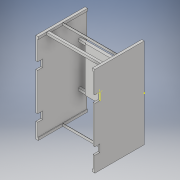
# Autodesk Inventor part: stand2.0
Saved by Autodesk Inventor 2019 (Build 230136000, 136)
## iProperties
Created: 2020-02-10
Part Number: stand2.0
Material: Generic
Document SubType Name: Modeling
Designer: Dell
Density: 1 g/cm^3
Appearance: Default
Author: Dell
Autodesk Inventor part; units mm, degrees
ref_plane "YZ Plane" through (0, 0, 0) normal (1, 0, 0) x (0, 1, 0)
ref_plane "XZ Plane" through (0, 0, 0) normal (0, 1, 0) x (-1, 0, 0)
ref_plane "XY Plane" through (0, 0, 0) normal (0, 0, 1) x (1, 0, 0)
sketch "Sketch1" plane through (0, 0, 0) normal (0, 0, 1) x (1, 0, 0)
  line L0 (-240, 365) -> (240, 365)
  line L1 (240, 365) -> (240, -365)
  line L2 (240, -365) -> (-240, -365)
  line L3 (-240, -365) -> (-240, 365)
  line L4 (-225, 345) -> (225, 345)
  line L5 (225, 345) -> (225, -345)
  line L6 (225, -345) -> (-225, -345)
  line L7 (-225, -345) -> (-225, 345)
  point P0 (0, 0)
  dimension "d0" = 480
  dimension "d1" = 730
  dimension "d2" = 450
  dimension "d3" = 690
  constraints: 16 end point, 4 parallel, 2 horizontal, 2 perpendicular
  measures "d0" distance of L1.end L2.end
  measures "d1" distance of L0.end L1.end
  measures "d2" distance of L5.end L6.end
  measures "d3" distance of L4.end L5.end
extrude "Extrusion1" add sketch "Sketch1" along normal blind 400
sketch "Sketch2" plane through (-240, 365, 0) normal (0, 1, 0) x (1, 0, 0)
  line L0 (20, 0) -> (20, -199)
  line L1 (20, 0) -> (219, 0) construction
  line L2 (20, -199) -> (460, -199)
  line L3 (460, -199) -> (460, 0)
  line L4 (15, 0) -> (465, 0) projected
  line L5 (465, -400) -> (15, -400) projected
  line L6 (20, -400) -> (20, -201)
  line L7 (15, 0) -> (15, -400) projected
  line L8 (20, -201) -> (460, -201)
  line L9 (20, -201) -> (460, -201) construction
  line L10 (460, -201) -> (460, -400)
  point P0 (240, 0)
  constraints: 16 end point, 3 perpendicular, 2 equal length, 2 horizontal, 2 point on line, 2 vertical, 1 parallel, 1 other
extrude "Extrusion2" cut sketch "Sketch2" against normal blind 740 contours L4 L3 L2 L0
sketch "Sketch3" plane through (-240, 365, 400) normal (0, 1, 0) x (1, 0, 0)
  line L0 (20, 0) -> (20, 199)
  line L1 (20, 199) -> (460, 199)
  line L2 (460, 199) -> (460, 0)
  line L3 (15, 0) -> (465, 0) projected
  point P0 (240, 400)
  dimension "d15" = 199
  dimension "d16" = 440
  constraints: 6 end point, 2 perpendicular, 1 point on line, 1 vertical
  measures "d15" distance of L0.start L0.end
  measures "d16" distance of L0.end L1.end
extrude "Extrusion3" cut sketch "Sketch3" against normal blind 740
sketch "Sketch8" plane through (-225, -345, 0) normal (1, 0, 0) x (0, 0, -1)
  line L0 (-50, 527.5) -> (-70, 527.5)
  line L1 (-70, 527.5) -> (-70, 507.5)
  line L2 (-70, 507.5) -> (-50, 507.5)
  line L3 (-50, 507.5) -> (-50, 527.5)
  point P0 (0, 345)
  point P1 (0, 345)
  constraints: 8 end point, 2 parallel, 1 coincident, 1 horizontal, 1 perpendicular
extrude "Extrusion6" add sketch "Sketch8" along normal blind 460
sketch "Sketch9" plane through (-225, -345, 0) normal (1, 0, 0) x (0, 0, -1)
  line L0 (-50, 182.5) -> (-70, 182.5)
  line L1 (-70, 182.5) -> (-70, 162.5)
  line L2 (-70, 162.5) -> (-50, 162.5)
  line L3 (-50, 162.5) -> (-50, 182.5)
  point P0 (0, 345)
  constraints: 8 end point, 2 parallel, 1 horizontal, 1 perpendicular
extrude "Extrusion7" add sketch "Sketch9" along normal blind 460
sketch "Sketch11" plane through (240, -365, 0) normal (1, 0, 0) x (0, 0, -1)
  line L0 (-400, 730) -> (-400, 0) projected
  line L1 (-400, 20) -> (-400, 710) projected
  line L2 (-400, 185.5) -> (-360, 185.5)
  line L3 (-360, 185.5) -> (-360, 125.5)
  line L4 (-360, 125.5) -> (-400, 125.5)
  line L5 (-400, 125.5) -> (-400, 185.5)
  point P0 (0, 365)
  point P1 (-400, 365)
  constraints: 8 end point, 2 parallel, 1 horizontal, 1 midpoint, 1 perpendicular, 1 point on line
extrude "Extrusion8" cut sketch "Sketch11" against normal blind 500
sketch "Sketch12" plane through (240, -365, 0) normal (1, 0, 0) x (0, 0, -1)
  line L0 (-400, 710) -> (-400, 185.5) projected
  line L1 (-400, 550.5) -> (-360, 550.5)
  line L2 (-360, 550.5) -> (-360, 490.5)
  line L3 (-360, 490.5) -> (-400, 490.5)
  line L4 (-400, 490.5) -> (-400, 550.5)
  point P0 (0, 365)
  point P1 (-400, 365)
  constraints: 8 end point, 2 parallel, 2 point on line, 1 horizontal, 1 perpendicular
extrude "Extrusion9" cut sketch "Sketch12" against normal blind 500
sketch "Sketch13" plane through (240, -365, 0) normal (1, 0, 0) x (0, 0, -1)
  line L0 (-360, 490.5) -> (-360, 550.5) projected
  point P0 (0, 365)
sketch "Sketch14" plane through (240, -365, 0) normal (1, 0, 0) x (0, 0, -1)
  point P0 (0, 365)
sketch "Sketch15" plane through (240, -365, 0) normal (1, 0, 0) x (0, 0, -1)
  point P0 (0, 365)
sketch "Sketch16" plane through (240, -365, 0) normal (1, 0, 0) x (0, 0, -1)
  point P0 (0, 365)
sketch "Sketch17" plane through (-225, -345, 0) normal (1, 0, 0) x (0, 0, -1)
  line L0 (-332.1423, 706.8149) -> (-312.1423, 706.8149)
  line L1 (-312.1423, 706.8149) -> (-312.1423, 686.8149)
  line L2 (-312.1423, 686.8149) -> (-332.1423, 686.8149)
  line L3 (-332.1423, 686.8149) -> (-332.1423, 706.8149)
  point P0 (0, 345)
  dimension "d43" = 20
  dimension "d44" = 20
  constraints: 8 end point, 2 parallel, 1 horizontal, 1 perpendicular
  measures "d43" distance of L1.end L2.end
  measures "d44" distance of L0.end L1.end
extrude "Extrusion10" add sketch "Sketch17" along normal blind 450
sketch "Sketch18" plane through (-225, 162.5, 70) normal (0, 0, 1) x (1, 0, 0)
  line L0 (0, 20) -> (450, 20) projected
  line L1 (0, -345) -> (450, -345) projected
  line L2 (60, 20) -> (380, 20)
  line L3 (380, 20) -> (380, -345)
  line L4 (380, -345) -> (60, -345)
  line L5 (60, -345) -> (60, 20)
  point P0 (225, -162.5)
  dimension "d47" = 320
  constraints: 8 end point, 2 parallel, 2 point on line, 1 horizontal, 1 perpendicular
  measures "d47" distance of L3.end L4.end
extrude "Extrusion11" add sketch "Sketch18" along normal blind 5
sketch "Sketch19" plane through (-225, 162.5, 75) normal (0, 0, 1) x (1, 0, 0)
  line L0 (175, -112.5) -> (275, -112.5)
  line L1 (275, -112.5) -> (275, -212.5)
  line L2 (275, -212.5) -> (175, -212.5)
  line L3 (175, -212.5) -> (175, -112.5)
  point P0 (225, -162.5)
  dimension "d50" = 100
  dimension "d51" = 100
  constraints: 8 end point, 2 parallel, 1 horizontal, 1 perpendicular
  measures "d50" distance of L1.end L2.end
  measures "d51" distance of L0.end L1.end
extrude "Extrusion12" add sketch "Sketch19" along normal blind 5
sketch "Sketch20" plane through (-225, 162.5, 80) normal (0, 0, 1) x (1, 0, 0)
  circle A0 centre (200, -162.5) radius 5.5
  point P0 (225, -162.5)
  dimension "d54" = 11
  constraints: 1 centre point
  measures "d54" diameter of A0
sketch "Sketch21" plane through (-225, 162.5, 80) normal (0, 0, 1) x (1, 0, 0)
  circle A0 centre (250, -162.5) radius 5.5
  point P0 (225, -162.5)
  dimension "d57" = 11
  constraints: 1 centre point
  measures "d57" diameter of A0
body "Solid1"
